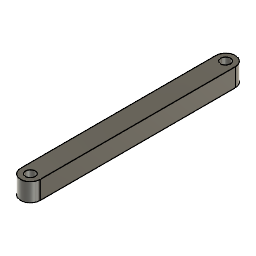
Prototyp (Autodesk Fusion 360 archive; units mm, degrees)
design "dl"
part number: 2026-03-17-22-02-21-073
Autodesk Fusion 360 part; units mm, degrees
sketch "Sketch1" plane through (0, 0, 0) normal (0, 0, 1) x (1, 0, 0)
  circle A0 centre (0, 140) radius 4
  circle A1 centre (0, -20) radius 4
  line L0 (8, 140) -> (8, -20)
  line L1 (-8, 140) -> (-8, -20)
  arc A2 (8, 140) -> (-8, 140) centre (0, 140) ccw
  arc A3 (-8, -20) -> (8, -20) centre (0, -20) ccw
  dimension "d1" = 160
  dimension "d4" = 8
  dimension "d5" = 8
  dimension "d7" = 16
  dimension "d8" = 16
  constraint concentric A1 A3
  constraint concentric A0 A2
  constraint tangent L0 A3
  constraint tangent L1 A3
  measures "d1" distance of A0.centre A1.centre
  measures "d4" diameter of A0
  measures "d5" diameter of A1
  measures "d7" diameter of A3
  measures "d8" diameter of A2
extrude "Extrude1" add sketch "Sketch1" along normal blind 25
extrude "Extrude2" cut 1 faces at (-6, 85.512, 25) along direction (0, 0, -1) blind 5
extrude "Extrude3" cut 1 faces at (-6, 85.512, 20) along direction (0, 0, -1) blind 5

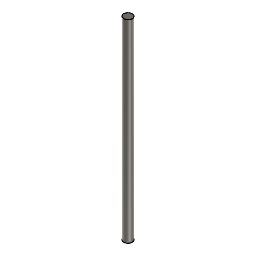
design "os"
part number: 2026-03-17-21-59-31-620
Autodesk Fusion 360 part; units mm, degrees
sketch "Sketch1" plane through (0, 0, 0) normal (0, 0, 1) x (1, 0, 0)
  circle A0 centre (0, 0) radius 4
  dimension "d1" = 8
  constraint coincident A0.centre origin
  measures "d1" diameter of A0
extrude "Extrude1" add sketch "Sketch1" along normal blind 180

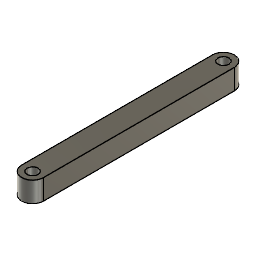
design "kr"
part number: 2026-03-17-22-22-28-821
Autodesk Fusion 360 part; units mm, degrees
sketch "Sketch1" plane through (0, 0, 0) normal (0, 0, 1) x (1, 0, 0)
  circle A0 centre (0, 90) radius 4
  circle A1 centre (0, -50) radius 4
  line L0 (8, 90) -> (8, -50)
  line L1 (-8, 90) -> (-8, -50)
  line L2 (0, -46) -> (0, -42)
  arc A2 (8, 90) -> (-8, 90) centre (0, 90) ccw
  arc A3 (-8, -50) -> (8, -50) centre (0, -50) ccw
  dimension "d1" = 140
  dimension "d2" = 8
  dimension "d3" = 16
  dimension "d4" = 8
  dimension "d5" = 16
  constraint vertical L2
  constraint concentric A0 A2
  constraint concentric A1 A3
  constraint tangent L0 A3
  constraint coincident A1 L2.start
  measures "d1" distance of A0.centre A1.centre
  measures "d2" diameter of A0
  measures "d3" diameter of A2
  measures "d4" diameter of A1
  measures "d5" diameter of A3
extrude "Extrude1" add sketch "Sketch1" along normal blind 15
